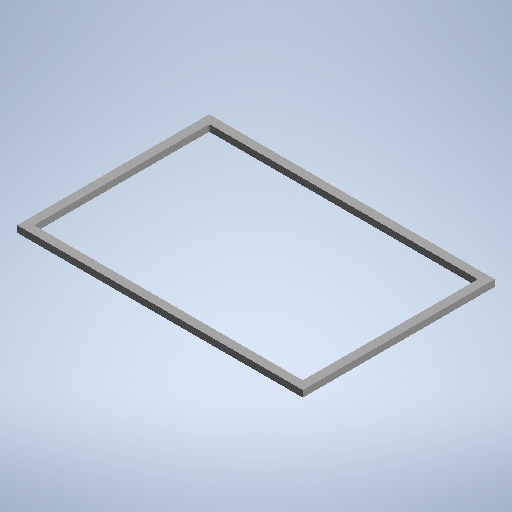
# Autodesk Inventor part: RT_TR_MC_001_TopPlate
Saved by Autodesk Inventor 2025.4 (Build 294407000, 407)
## iProperties
Created: 2026-08-10
Part Number: RT_TR_MC_001_TopPlate
Material: Générique
Document SubType Name: Modeling
Designer: louis
Density: 1 g/cm^3
Appearance: Par défaut
Author: louis
Autodesk Inventor part; units mm, degrees
ref_plane "YZ Plane" through (0, 0, 0) normal (1, 0, 0) x (0, 1, 0)
ref_plane "XZ Plane" through (0, 0, 0) normal (0, 1, 0) x (-1, 0, 0)
ref_plane "XY Plane" through (0, 0, 0) normal (0, 0, 1) x (1, 0, 0)
sketch "Sketch2" plane through (0, 0, 0) normal (0, 0, 1) x (1, 0, 0)
  line L0 (-305, -205) -> (305, -205)
  line L1 (305, -205) -> (305, 205)
  line L2 (305, 205) -> (-305, 205)
  line L3 (-305, 205) -> (-305, -205)
  line L4 (-305, -205) -> (305, 205) construction
  line L5 (305, -205) -> (-305, 205) construction
  point P0 (0, 0)
  dimension "d0" = 610
  dimension "d1" = 410
  constraints: 12 end point, 2 midpoint, 2 parallel, 1 horizontal, 1 perpendicular
  measures "d0" distance of L2.end L1.end
  measures "d1" distance of L1.end L0.end
extrude "Extrusion1" add sketch "Sketch2" along normal blind 14
sketch "Sketch3" plane through (0, 0, 14) normal (0, 0, 1) x (1, 0, 0)
  line L0 (-283, -187) -> (283, -187)
  line L1 (287, -183) -> (287, 183)
  line L2 (283, 187) -> (-283, 187)
  line L3 (-287, 183) -> (-287, -183)
  line L4 (-287, -187) -> (287, 187) construction
  line L5 (287, -187) -> (-287, 187) construction
  arc A0 (-283, 187) -> (-287, 183) centre (-283, 183) ccw
  arc A1 (287, 183) -> (283, 187) centre (283, 183) ccw
  arc A2 (283, -187) -> (287, -183) centre (283, -183) ccw
  arc A3 (-287, -183) -> (-283, -187) centre (-283, -183) ccw
  point P0 (0, 0)
  dimension "d4" = 374
  dimension "d5" = 574
  dimension "d6" = 4
  constraints: 12 end point, 8 point on circle, 8 point on line, 8 tangent, 4 centre point, 3 equal radius, 2 midpoint, 2 parallel, 1 horizontal, 1 perpendicular
  measures "d4" distance of L5.end L4.start
  measures "d5" distance between parallel lines of L1 L3
  measures "d6" radius of A0
extrude "Extrusion2" cut sketch "Sketch3" against normal through all
body "Solid1"
